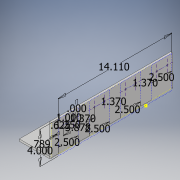
# Autodesk Inventor part: ubracket
Saved by Autodesk Inventor 2017 (Build 210142000, 142)
## iProperties
Created: 2018-03-08
Part Number: ubracket
Material: Generic
Document SubType Name: Sheet Metal
Designer: Zara
Density: 1 g/cm^3
Sheet Metal Rule: Default
Appearance: Default
Author: Zara
Autodesk Inventor part; units mm, degrees
ref_plane "YZ Plane" through (0, 0, 0) normal (1, 0, 0) x (0, 1, 0)
ref_plane "XZ Plane" through (0, 0, 0) normal (0, 1, 0) x (-1, 0, 0)
ref_plane "XY Plane" through (0, 0, 0) normal (0, 0, 1) x (1, 0, 0)
sketch "Sketch1" plane through (0, 0, 0) normal (0, 1, 0) x (-1, 0, 0)
  line L0 (59.2667, 296.3333) -> (-42.3333, 296.3333)
  line L1 (-42.3333, 296.3333) -> (-42.3333, -84.6667)
  line L2 (-42.3333, -84.6667) -> (59.2667, -84.6667)
  line L3 (59.2667, -84.6667) -> (59.2667, 296.3333)
  point P0 (0, 0)
  dimension "d0" = 101.6
  dimension "d1" = 381
  measures "d0" distance of L1.end L2.end
  measures "d1" distance of L0.end L1.end
extrude "Plate1" add sketch "Sketch1" along normal blind 6.35
sketch "Sketch2" plane through (35.9833, 0, -84.6667) normal (1, 0, 0) x (0, 1, 0)
  line L0 (0, 381) -> (0, 0)
  line L1 (0, 0) -> (101.6, 0)
  line L2 (101.6, 0) -> (101.6, 381)
  line L3 (101.6, 381) -> (0, 381)
  constraints: 6 end point, 1 horizontal, 1 perpendicular, 1 vertical
edge flange "Flange1" height 101.6 angle 90 thickness 6.35 bend radius 0.0254 thickness toward (1, 0, 0) relief straight relief width 6.35 relief depth 3.175 edges at (42.3333, 6.35, 105.8333) wall of the first edge with corners at (35.9833, 0, 296.3333) (35.9833, 0, -84.6667) (35.9833, 101.6, -84.6667) (35.9833, 101.6, 296.3333)
bend "Bend1"
corner "Corner1"
sketch "Sketch3" plane through (42.3333, 101.6, 296.3333) normal (1, 0, 0) x (0, 0, -1)
  line L0 (20.0406, 0) -> (378.4346, 0) construction
  line L1 (378.4346, 0) -> (378.4346, -101.6) construction
  line L2 (378.4346, -101.6) -> (20.0406, -101.6) construction
  line L3 (20.0406, -101.6) -> (20.0406, 0) construction
  line L4 (0, -95.2246) -> (0, 0) construction
  line L5 (0, 0) -> (381, 0) construction
  line L6 (20.0406, 0) -> (83.5406, 0) construction
  line L7 (83.5406, 0) -> (83.5406, -95.25) construction
  line L8 (83.5406, -95.25) -> (20.0406, -95.25) construction
  line L9 (20.0406, -95.25) -> (20.0406, 0) construction
  line L10 (118.3386, 0) -> (181.8386, 0) construction
  line L11 (181.8386, 0) -> (181.8386, -95.25) construction
  line L12 (181.8386, -95.25) -> (118.3386, -95.25) construction
  line L13 (118.3386, -95.25) -> (118.3386, 0) construction
  line L14 (216.6366, 0) -> (280.1366, 0) construction
  line L15 (280.1366, 0) -> (280.1366, -95.25) construction
  line L16 (280.1366, -95.25) -> (216.6366, -95.25) construction
  line L17 (216.6366, -95.25) -> (216.6366, 0) construction
  line L18 (314.9346, 0) -> (378.4346, 0) construction
  line L19 (378.4346, 0) -> (378.4346, -95.25) construction
  line L20 (378.4346, -95.25) -> (314.9346, -95.25) construction
  line L21 (314.9346, -95.25) -> (314.9346, 0) construction
  line L22 (35.9156, -25.4) -> (67.6656, -25.4) construction
  line L23 (134.4168, -25.4) -> (166.1668, -25.4) construction
  line L24 (232.918, -25.4) -> (264.668, -25.4) construction
  line L25 (331.4192, -25.4) -> (363.1692, -25.4) construction
  point P0 (296.3333, -101.6)
  dimension "d13" = 358.394
  dimension "d14" = 20.0406
  dimension "d15" = 101.6
  dimension "d16" = 0
  dimension "d17" = 63.5
  dimension "d18" = 63.5
  dimension "d19" = 34.798
  dimension "d20" = 63.5
  dimension "d21" = 34.798
  dimension "d22" = 63.5
  dimension "d23" = 34.798
  dimension "d24" = 25.4
  dimension "d25" = 31.75
  dimension "d26" = 15.875
  dimension "d36" = 98.5012
  constraints: 48 end point, 10 parallel, 7 horizontal, 5 perpendicular, 3 point on line, 1 collinear, 8 other
  measures "d13" distance of L0.start L0.end
  measures "d14" distance between parallel lines of L4 L3
  measures "d15" distance of L2.end L0.start
  measures "d16" distance between parallel lines of L5 L0
  measures "d17" distance of L7.end L8.end
  measures "d18" distance of L11.end L12.end
  measures "d19" distance between parallel lines of L7 L13
  measures "d20" distance of L15.end L16.end
  measures "d21" distance between parallel lines of L11 L17
  measures "d22" distance between parallel lines of L19 L21
  measures "d23" distance between parallel lines of L15 L21
  measures "d24" distance between parallel lines of L6 L22
  measures "d25" distance of L22.start L22.end
  measures "d26" distance from line of L9 L22.start
  measures "d36" distance of L22.start L23.start
hole "Hole1" at (42.3333, 76.2, 260.4177) at (42.3333, 76.2, 228.6677) at (42.3333, 76.2, 130.1665) at (42.3333, 76.2, 161.9165) at (42.3333, 76.2, 63.4153) at (42.3333, 76.2, 31.6653) at (42.3333, 76.2, -35.0859) at (42.3333, 76.2, -66.8359) direction (-1, 0, 0) diameter 3.9624 depth 13.6144 tip angle 118 thread size "10-32 UNF" class "2B" standard "ANSI Unified Screw Threads"
sketch "Sketch4" plane through (0, 6.35, 0) normal (0, 1, 0) x (1, 0, 0)
  line L0 (-59.2667, -296.3333) -> (-59.2667, 84.6667) projected
  line L1 (-59.2667, 84.6667) -> (35.9579, 84.6667) projected
  line L2 (42.3333, -296.3333) -> (42.3333, 84.6667) projected
  line L3 (35.9579, -296.3333) -> (-59.2667, -296.3333) projected
  point P0 (7.4083, 59.2667)
  point P1 (7.4083, -16.9333)
  point P2 (7.4083, -67.7333)
  point P3 (7.4083, -143.9333)
  point P4 (7.4083, -194.7333)
  point P5 (7.4083, -270.9333)
  dimension "d42" = 25.4
  dimension "d45" = 76.2
  dimension "d58" = 34.925
  dimension "d59" = 34.925
  dimension "d60" = 50.8
  dimension "d61" = 76.2
  dimension "d62" = 50.8
  dimension "d63" = 76.2
  dimension "d64" = 25.4
  dimension "d65" = 34.925
  dimension "d66" = 34.925
  dimension "d67" = 34.925
  measures "d42" distance from line of point (7.408, 59.267) L1
  measures "d45" distance of point (7.408, 59.267) point (7.408, -16.933)
  measures "d58" distance from line of L2 point (7.408, 59.267)
  measures "d59" distance from line of L2 point (7.408, -16.933)
  measures "d60" distance of point (7.408, -67.733) point (7.408, -16.933)
  measures "d61" distance of point (7.408, -143.933) point (7.408, -67.733)
  measures "d62" distance of point (7.408, -194.733) point (7.408, -143.933)
  measures "d63" distance of point (7.408, -270.933) point (7.408, -194.733)
  measures "d64" distance from line of L3 point (7.408, -270.933)
  measures "d65" distance from line of L2 point (7.408, -67.733)
  measures "d66" distance from line of L2 point (7.408, -143.933)
  measures "d67" distance from line of L2 point (7.408, -194.733)
hole "Hole2" at (7.4083, 6.35, -59.2667) at (7.4083, 6.35, 16.9333) at (7.4083, 6.35, 67.7333) at (7.4083, 6.35, 143.9333) at (7.4083, 6.35, 194.7333) at (7.4083, 6.35, 270.9333) direction (0, -1, 0) diameter 3.9624 depth 13.6144 tip angle 118 thread size "10-32 UNF" class "2B" standard "ANSI Unified Screw Threads"
equation "\"d3\" = BendReliefWidth"
equation "\"d4\" = BendReliefDepth"
equation "\"d5\" = MinimumRemnant"
equation "\"d6\" = BendRadius"
equation "\"d10\" = CornerReliefSize"
equation "\"d11\" = GapSize"
equation "\"d12\" = JacobiRadiusSize"
equation "\"BendRadius\" = Thickness"
equation "\"BendReliefWidth\" = Thickness"
equation "\"BendReliefDepth\" = 0.5 * Thickness"
equation "\"CornerReliefSize\" = 4 * Thickness"
equation "\"MinimumRemnant\" = 2 * Thickness"
equation "\"TransitionRadius\" = BendRadius"
equation "\"JacobiRadiusSize\" = Thickness"
equation "\"GapSize\" = Thickness"
equation "\"d2\" = BendRadius"
equation "\"Thickness\" = 6.35"
body "Solid1"
